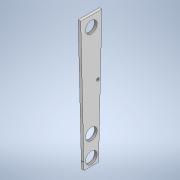
# Autodesk Inventor part: Intake - Side Panel
Saved by Autodesk Inventor 2020 (Build 240168000, 168)
## iProperties
Created: 2020-02-06
Part Number: Intake - Side Panel
Material: Generic
Document SubType Name: Modeling
Designer: aidan
Density: 1 g/cm^3
Appearance: Default
Author: aidan
Autodesk Inventor part; units mm, degrees
ref_plane "YZ Plane" through (0, 0, 0) normal (1, 0, 0) x (0, 1, 0)
ref_plane "XZ Plane" through (0, 0, 0) normal (0, 1, 0) x (-1, 0, 0)
ref_plane "XY Plane" through (0, 0, 0) normal (0, 0, 1) x (1, 0, 0)
sketch "Sketch1" plane through (0, 0, 0) normal (1, 0, 0) x (0, 1, 0)
  line L0 (0, -38.1) -> (254, -44.45)
  line L1 (254, -44.45) -> (254, 6.35)
  line L2 (254, 6.35) -> (0, 0)
  line L3 (0, 0) -> (0, -38.1)
  arc A0 (254, -44.45) -> (254, 6.35) centre (254, -19.05) ccw
  circle A1 centre (254, -19.05) radius 14.2875
  circle A2 centre (25.4, -19.05) radius 14.2875
  point P0 (0, -19.05)
  point P1 (254, -33.3375)
  point P2 (254, -4.7625)
  dimension "d3" = 50.8
  dimension "d4" = 38.1
  dimension "d5" = 28.575
  dimension "d6" = 28.575
  dimension "d8" = 228.6
  dimension "d9" = 254
  constraints: 8 end point, 3 centre point, 3 coincident, 3 point on circle, 2 horizontal alignment, 2 midpoint, 1 parallel, 1 point on line, 1 vertical
  measures "d3" distance of L0.end L1.end
  measures "d4" distance of L0.start L2.end
  measures "d5" diameter of A1
  measures "d6" diameter of A2
  measures "d8" distance of A2.centre point (254, -19.05)
  measures "d9" distance between parallel lines of L3 L1
extrude "Extrusion1" add sketch "Sketch1" against normal blind 6.35 contours L3 L2 L1 A1 L0 | L1 A1 A0
sketch "Sketch3" plane through (-6.35, 0, 0) normal (-1, 0, 0) x (0, 0, 1)
  line L0 (-38.1, 0) -> (0, 0) projected
  line L1 (0, 0) -> (-0.635, -25.4)
  line L2 (-44.45, 254) -> (-38.1, 0) projected
  line L3 (-38.1, 0) -> (-37.465, -25.4)
  line L4 (0, 0) -> (6.35, 254) projected
  line L5 (-37.465, -25.4) -> (-0.635, -25.4)
  arc A0 (-37.465, -25.4) -> (-0.635, -25.4) centre (-19.05, -25.4) ccw
  circle A1 centre (-19.05, -25.4) radius 14.2875
  dimension "d12" = 25.4
  dimension "d13" = 28.575
  constraints: 6 end point, 2 centre point, 2 collinear, 2 point on circle, 1 coincident, 1 midpoint, 1 parallel
  measures "d12" distance between parallel lines of L0 L5
  measures "d13" diameter of A1
extrude "Extrusion2" add sketch "Sketch3" against normal blind 6.35 contours L0 L1 L5 A1 L3 | L5 A1 A0
sketch "Sketch4" plane through (-6.35, 0, 0) normal (-1, 0, 0) x (0, 0, 1)
  line L0 (6.35, 254) -> (-0.635, -25.4) projected
  line L1 (-0.635, -25.4) -> (-1.0954, -43.815)
  line L2 (-37.465, -25.4) -> (-44.45, 254) projected
  line L3 (-37.465, -25.4) -> (-37.0046, -43.815)
  arc A0 (-37.465, -25.4) -> (-0.635, -25.4) centre (-19.05, -25.4) ccw projected
  line L4 (-1.0954, -43.815) -> (-37.0046, -43.815)
  line L5 (6.35, 254) -> (6.985, 279.4)
  line L6 (-44.45, 254) -> (-45.085, 279.4)
  arc A1 (6.35, 254) -> (-44.45, 254) centre (-19.05, 254) ccw projected
  line L7 (6.985, 279.4) -> (-45.085, 279.4)
  point P0 (0, 0)
  point P1 (-19.05, -43.815)
  point P2 (-19.05, -43.815)
  point P3 (-19.05, 279.4)
  point P4 (-19.05, 279.4)
  point P5 (-19.05, -43.815)
  point P6 (-0.658, -26.3202)
  point P7 (-37.442, -26.3202)
  point P8 (-19.05, 279.4)
  constraints: 12 end point, 4 collinear, 4 horizontal alignment, 4 point on circle, 2 horizontal
extrude "Extrusion3" add sketch "Sketch4" against normal blind 6.35 contours A1 L7 L5 | A1 L6 L7 | L1 L4 A0 | L4 L3 A0
sketch "Sketch5" plane through (-6.35, 0, 0) normal (-1, 0, 0) x (0, 0, 1)
  circle A0 centre (-35.0976, 133.985) radius 3.175
  line L0 (-37.0046, -43.815) -> (-1.0954, -43.815) projected
  line L1 (-0.635, -25.4) -> (6.985, 279.4) projected
  line L2 (-45.085, 279.4) -> (-37.465, -25.4) projected
  point P0 (0, 0)
  dimension "d18" = 6.35
  dimension "d19" = 177.8
  dimension "d28" = 6.35
  constraints: 1 centre point
  measures "d18" diameter of A0
  measures "d19" distance from line of L0 A0.centre
  measures "d28" distance from line of L2 A0.centre
hole "Hole1" at (-6.35, 133.985, -35.0976) direction (1, 0, 0) diameter 6.35 depth 38.1 tip angle 118
body "Solid1"
